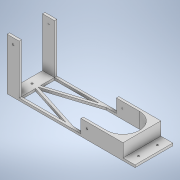
# Autodesk Inventor part: frame
Saved by Autodesk Inventor 2020 (Build 240168000, 168)
## iProperties
Created: 2020-02-29
Part Number: frame
Material: Типовые
Document SubType Name: Modeling
Designer: CSS38
Density: 1 g/cm^3
Appearance: По умолчанию
Author: CSS38
Autodesk Inventor part; units mm, degrees
ref_plane "YZ Plane" through (0, 0, 0) normal (1, 0, 0) x (0, 1, 0)
ref_plane "XZ Plane" through (0, 0, 0) normal (0, 1, 0) x (-1, 0, 0)
ref_plane "XY Plane" through (0, 0, 0) normal (0, 0, 1) x (1, 0, 0)
sketch "Эскиз1" plane through (0, 0, 0) normal (0, 1, 0) x (-1, 0, 0)
  line L0 (-53.25, 15.75) -> (53.25, 15.75)
  line L1 (53.25, 15.75) -> (53.25, -15.75)
  line L2 (53.25, -15.75) -> (-53.25, -15.75)
  line L3 (-53.25, -15.75) -> (-53.25, 15.75)
  line L4 (-53.25, 15.75) -> (53.25, -15.75) construction
  line L5 (53.25, 15.75) -> (-53.25, -15.75) construction
  line L6 (-43.25, -13.75) -> (0, -13.75)
  line L7 (43.25, -13.75) -> (43.25, -2.0986)
  line L8 (43.25, 13.75) -> (6.6012, 13.75)
  line L9 (-43.25, 13.75) -> (-43.25, -13.75)
  line L10 (0, -22.05) -> (0, 22.05) construction
  line L11 (0, -15.75) -> (0, -13.75) construction
  line L12 (0, 13.75) -> (0, 15.75) construction
  line L13 (0, -13.75) -> (43.25, 0)
  line L14 (43.25, 0) -> (0, 13.75)
  line L15 (6.6012, 13.75) -> (43.25, 2.0986)
  line L16 (43.25, -2.0986) -> (6.6012, -13.75)
  line L17 (43.25, -2.0986) -> (43.25, 2.0986) construction
  line L18 (43.25, 2.0986) -> (43.25, 13.75)
  line L19 (6.6012, -13.75) -> (43.25, -13.75)
  line L20 (0, -13.75) -> (6.6012, -13.75) construction
  line L21 (6.6012, 13.75) -> (0, 13.75) construction
  line L22 (0, 13.75) -> (-43.25, 13.75)
  line L23 (43.25, -2.0986) -> (42.644, -0.1926) construction
  line L24 (43.25, 2.0986) -> (42.644, 0.1926) construction
  point P0 (0, 0)
  point P1 (0, 0)
  dimension "d0" = 106.5
  dimension "d5" = 10
  dimension "d24" = 27.5
  dimension "d28" = 10
  dimension "d29" = 2
  constraints: 48 end point, 16 parallel, 16 perpendicular, 4 equal length, 4 midpoint, 4 point on line, 2 collinear, 1 coincident, 1 horizontal
  measures "d0" distance of L1.end L2.end
  measures "d5" distance between parallel lines of L9 L3
  measures "d24" distance of L9.start L6.start
  measures "d28" distance between parallel lines of L1 L7
  measures "d29" distance of L11.start L6.end
extrude "Выдавливание1" add sketch "Эскиз1" along normal blind 2
sketch "Эскиз2" plane through (0, 0, 0) normal (0, 1, 0) x (-1, 0, 0)
  line L0 (-43.25, -15.75) -> (-43.25, 15.75)
  line L1 (53.25, 15.75) -> (-53.25, 15.75) projected
  line L2 (-53.25, 15.75) -> (-53.25, -15.75) projected
  line L3 (0, -13.75) -> (-43.25, -13.75) construction
  line L4 (-41.25, -13.75) -> (-41.25, 13.75) construction
  line L5 (6.6012, 13.75) -> (43.25, 13.75) construction
  line L6 (-41.25, -13.75) -> (-27.5, -13.75) construction
  line L7 (-8.25, -13.75) -> (-8.25, -15.75)
  line L8 (-53.25, -15.75) -> (53.25, -15.75) projected
  line L9 (-8.25, -15.75) -> (-43.25, -15.75)
  line L10 (-43.25, 15.75) -> (-8.25, 15.75)
  line L11 (-8.25, 13.75) -> (-27.5, 13.75)
  line L12 (-8.25, 13.75) -> (-8.25, 15.75)
  arc A0 (-27.5, 13.75) -> (-27.5, -13.75) centre (-27.5, 0) ccw
  line L13 (-27.5, -13.75) -> (-8.25, -13.75)
  line L14 (-27.5, 13.75) -> (-41.25, 13.75) construction
  line L15 (-43.25, -13.75) -> (-43.25, 13.75) projected
  point P0 (0, 0)
  point P1 (43.25, -13.75)
  point P2 (-43.25, -15.75)
  dimension "d13" = 2
  dimension "d14" = 33
  constraints: 20 end point, 7 point on line, 5 tangent, 4 collinear, 3 perpendicular, 3 vertical, 2 point on circle, 1 centre point
  measures "d13" distance between parallel lines of L0 L4
  measures "d14" distance of L4.start L7.start
extrude "Выдавливание2" add sketch "Эскиз2" along normal blind 13 contours L0 L1 L12 L11 A0 L13 L7 L8
sketch "Эскиз3" plane through (0, 2, 0) normal (0, 1, 0) x (1, 0, 0)
  line L0 (-43.25, 13.75) -> (-53.25, 13.75)
  line L1 (-53.25, 13.75) -> (-53.25, 15.75)
  line L2 (-53.25, 15.75) -> (-43.25, 15.75)
  line L3 (-43.25, 15.75) -> (-43.25, 13.75)
  line L4 (-53.25, 15.75) -> (-53.25, -15.75) construction
  line L5 (-53.25, -15.75) -> (-43.25, -15.75)
  line L6 (-43.25, -15.75) -> (-43.25, -13.75)
  line L7 (-43.25, -13.75) -> (-53.25, -13.75)
  line L8 (-53.25, -13.75) -> (-53.25, -15.75)
  point P0 (0, 0)
  point P1 (8.25, -13.75)
  constraints: 16 end point, 4 parallel, 2 coincident, 2 horizontal, 2 perpendicular
extrude "Выдавливание3" add sketch "Эскиз3" along normal blind 41
sketch "Эскиз4" plane through (-53.25, 0, 15.75) normal (0, 0, 1) x (1, 0, 0)
  line L0 (10, 43) -> (0, 43) construction
  line L1 (0, 43) -> (10, 43) construction
  line L2 (10, 43) -> (10, 33) construction
  line L3 (10, 33) -> (0, 33) construction
  line L4 (0, 33) -> (0, 43) construction
  line L5 (106.5, 0) -> (0, 0) construction
  line L6 (0, 0) -> (0, 43) construction
  line L7 (10, 43) -> (10, 2) construction
  line L8 (10, 2) -> (61.5, 2) construction
  line L9 (61.5, 2) -> (61.5, 13) construction
  line L10 (61.5, 13) -> (96.5, 13) construction
  line L11 (96.5, 13) -> (96.5, 2) construction
  line L12 (96.5, 2) -> (106.5, 2) construction
  line L13 (106.5, 2) -> (106.5, 0) construction
  line L14 (10, 2) -> (10, 43) construction
  line L15 (0, 0) -> (0, 43) construction
  line L16 (10, 33) -> (0, 43) construction
  line L17 (10, 43) -> (0, 33) construction
  circle A0 centre (5, 38) radius 0.5
  line L18 (61.5, 13) -> (71.5, 13) construction
  line L19 (71.5, 13) -> (71.5, 3) construction
  line L20 (71.5, 3) -> (61.5, 3) construction
  line L21 (61.5, 3) -> (61.5, 13) construction
  line L22 (71.5, 13) -> (61.5, 3) construction
  line L23 (61.5, 2) -> (61.5, 13) construction
  line L24 (61.5, 13) -> (71.5, 3) construction
  circle A1 centre (66.5, 8) radius 0.5
  line L25 (0, 43) -> (10, 43) projected
  point P0 (53.25, 0)
  dimension "d19" = 1
  dimension "d20" = 10
  dimension "d21" = 1
  constraints: 24 end point, 5 perpendicular, 4 parallel, 2 centre point, 2 horizontal, 2 midpoint, 1 collinear
  measures "d19" diameter of A0
  measures "d20" distance of L19.end L20.end
  measures "d21" diameter of A1
hole "Отверстие1" at (-48.25, 38, 15.75) at (13.25, 8, 15.75) direction (0, 0, -1) diameter 1 depth 15.75 countersink diameter 1.5 countersink angle 90
mirror "Зеркальное отражение1" about plane through (0, 0, 0) normal (0, 0, 1) of "Отверстие1"
sketch "Эскиз5" plane through (0, 2, 0) normal (0, 1, 0) x (1, 0, 0)
  line L0 (8.25, 13.75) -> (8.25, 15.75) construction
  line L1 (-43.25, 15.75) -> (8.25, 15.75) construction
  line L2 (-53.25, 15.75) -> (-43.25, 15.75) construction
  line L3 (-53.25, 13.75) -> (-53.25, 15.75) construction
  line L4 (-43.25, 13.75) -> (-53.25, 13.75) construction
  line L5 (-43.25, 13.75) -> (-43.25, 2.0986) construction
  line L6 (-43.25, 2.0986) -> (-6.6012, 13.75) construction
  line L7 (-6.6012, 13.75) -> (-43.25, 13.75) construction
  line L8 (8.25, 13.75) -> (0, 13.75) construction
  line L9 (27.5, 13.75) -> (8.25, 13.75) construction
  arc A0 (27.5, -13.75) -> (27.5, 13.75) centre (27.5, 0) ccw construction
  line L10 (8.25, -13.75) -> (27.5, -13.75) construction
  line L11 (8.25, -15.75) -> (8.25, -13.75) construction
  line L12 (8.25, -15.75) -> (-43.25, -15.75) construction
  line L13 (-43.25, -13.75) -> (-43.25, -15.75) construction
  line L14 (-43.25, -13.75) -> (-6.6012, -13.75) construction
  line L15 (-6.6012, -13.75) -> (-43.25, -2.0986) construction
  line L16 (-43.25, -2.0986) -> (-43.25, -13.75) construction
  line L17 (8.25, 15.75) -> (43.25, 15.75) construction
  line L18 (43.25, 15.75) -> (43.25, -15.75) construction
  line L19 (53.25, -15.75) -> (43.25, -15.75) construction
  line L20 (53.25, 15.75) -> (53.25, -15.75) construction
  line L21 (43.25, 15.75) -> (53.25, 15.75) construction
  line L22 (-43.25, 15.75) -> (-43.25, 13.75) construction
  line L23 (-53.25, -13.75) -> (-53.25, 13.75) construction
  line L24 (-53.25, -15.75) -> (-53.25, -13.75) construction
  line L25 (-43.25, -15.75) -> (-53.25, -15.75) construction
  line L26 (0, 13.75) -> (-43.25, 0) construction
  line L27 (-43.25, 0) -> (0, -13.75) construction
  line L28 (0, -13.75) -> (8.25, -13.75) construction
  line L29 (43.25, -15.75) -> (8.25, -15.75) construction
  line L30 (-53.25, -13.75) -> (-43.25, -13.75) construction
  line L31 (53.25, 15.75) -> (-53.25, 15.75) construction
  line L32 (-53.25, 15.75) -> (-43.25, -15.75) construction
  line L33 (-53.25, -15.75) -> (53.25, -15.75) construction
  line L34 (-53.25, -15.75) -> (-43.25, 15.75) construction
  line L35 (53.25, 15.75) -> (43.25, 0) construction
  line L36 (43.25, 15.75) -> (53.25, 0) construction
  line L37 (53.25, -15.75) -> (53.25, 15.75) construction
  line L38 (53.25, 0) -> (43.25, -15.75) construction
  line L39 (53.25, -15.75) -> (43.25, 0) construction
  circle A1 centre (-48.25, 0) radius 0.5
  circle A2 centre (48.25, 7.875) radius 0.5
  circle A3 centre (48.25, -7.875) radius 0.5
  point P0 (0, 0)
  dimension "d37" = 1
  constraints: 12 end point, 5 midpoint, 3 centre point, 2 equal radius, 2 parallel
  measures "d37" diameter of A1
hole "Отверстие2" at (-48.25, 2, 0) at (48.25, 2, 7.875) at (48.25, 2, -7.875) direction (0, -1, 0) diameter 1 end through all countersink diameter 1.5 countersink angle 90
